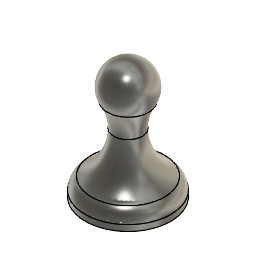
pion (Autodesk Fusion 360 design; units mm, degrees)
part number: 2026-06-29-11-37-21-556
Autodesk Fusion 360 part; units mm, degrees
note: some values were not read from the file. Set by a fixed rule: which sketch regions a step uses.
sketch "Esquisse1" plane through (0, 0, 0) normal (0, 1, 0) x (1, 0, 0)
  line L0 (0, 0) -> (9, 0)
  line L1 (3, -6) -> (3, -16)
  circle A0 centre (0, -20) radius 5
  line L2 (0, 0) -> (0, -25)
  line L3 (0, 0) -> (4.1, 0)
  line L4 (4.1, 0) -> (4.1, -3.2)
  line L5 (4.1, -3.2) -> (0, -3.2)
  line L6 (0, -3.2) -> (0, 0)
  line L7 (9, 0) -> (9, -3)
  line L8 (9, -3) -> (3, -6)
  dimension "d2" = 9
  dimension "d3" = 6
  dimension "d4" = 6
  dimension "d5" = 10
  dimension "d6" = 25
  dimension "d9" = 4.1
  dimension "d10" = 3.2
  dimension "d11" = 3
  constraint coincident L0.start L2.start
  constraint horizontal L0
  constraint vertical L1
  constraint coincident L1.end A0
  constraint coincident A0 L2.end
  constraint perpendicular L0 L2
  constraint coincident A0.centre L2
  constraint horizontal L3
  constraint vertical L4
  constraint horizontal L5
  constraint vertical L6
  constraint perpendicular L0 L7
  measures "d2" distance of L0.start L0.end
  measures "d3" distance of L0 L1.start
  measures "d4" horizontal distance of L0.end L1.start
  measures "d5" diameter of A0
  measures "d6" distance of L0.start L2.end
  measures "d9" distance of L4.end L5.end
  measures "d10" distance of L3.end L4.end
  measures "d11" distance of L0.end L7.end
revolve "Révolution1" add sketch "Esquisse1" angle 360 about axis through (0, 0, 0) along (0, 0, 1) contours L0 L1 A0 L2 L4 L5 L7 L8 | A0 L2 picked at (1.795, -18.9331)
fillet "Congé1" radius 10.5 1 faces at (2.9963, -0.1495, 9.3333)
fillet "Congé2" radius 3 1 edges at (-8.3909, -3.2545, 3)
